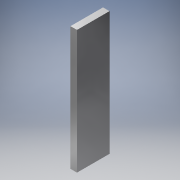
# Autodesk Inventor part: frame_front
Saved by Autodesk Inventor 2018 (Build 220112000, 112)
## iProperties
Created: 2018-05-23
Part Number: frame_front
Material: アルミニウム 6061
Document SubType Name: Sheet Metal
Designer: NaMACHAN
Density: 2.7 g/cm^3
Sheet Metal Rule: 2mmAl
Appearance: アルミニウム - フラット
Author: NaMACHAN
Autodesk Inventor part; units mm, degrees
ref_plane "YZ Plane" through (0, 0, 0) normal (1, 0, 0) x (0, 1, 0)
ref_plane "XZ Plane" through (0, 0, 0) normal (0, 1, 0) x (-1, 0, 0)
ref_plane "XY Plane" through (0, 0, 0) normal (0, 0, 1) x (1, 0, 0)
sketch "スケッチ1" plane through (0, 0, 0) normal (1, 0, 0) x (0, 1, 0)
  line L0 (0, 0) -> (0, -38)
  line L1 (0, -38) -> (-10, -38)
  line L2 (-10, -38) -> (-10, 0)
  line L3 (-10, 0) -> (0, 0)
  dimension "d0" = 38
  dimension "d2" = 10
  measures "d0" distance of L0.start L0.end
  measures "d2" distance of L0.end L1.end
extrude "プレート1" add sketch "スケッチ1" along normal blind 2
sketch "スケッチ14" plane through (-2, 2, -38) normal (0, 1, 0) x (-1, 0, 0)
  line L0 (0, 38) -> (0, 0)
  line L1 (0, 0) -> (8, 0)
  line L2 (8, 0) -> (8, 38)
  line L3 (8, 38) -> (0, 38)
  constraints: 6 end point, 1 horizontal, 1 perpendicular, 1 vertical
edge flange "フランジ1" height 12 angle 90 thickness 2 bend radius 2 thickness toward (0, 1, 0) relief tear relief width 2 relief depth 1 edges at (0, 0, -19) wall of the first edge with corners at (-2, 2, 0) (-2, 2, -38) (-10, 2, -38) (-10, 2, 0)
bend "曲げ26"
corner "コーナー1"
sketch "スケッチ15" plane through (-2, -12, 0) normal (0, -1, 0) x (1, 0, 0)
  line L0 (0, -38) -> (0, 0)
  line L1 (0, 0) -> (-8, 0)
  line L2 (-8, 0) -> (-8, -38)
  line L3 (-8, -38) -> (0, -38)
  constraints: 6 end point, 1 horizontal, 1 perpendicular, 1 vertical
edge flange "フランジ2" height 12 angle 90 thickness 2 bend radius 2 thickness toward (0, -1, 0) relief tear relief width 2 relief depth 1 edges at (0, -10, -19) wall of the first edge with corners at (-2, -12, -38) (-2, -12, 0) (-10, -12, 0) (-10, -12, -38)
bend "曲げ27"
corner "コーナー2"
sketch "スケッチ16" plane through (-10, 4, 0) normal (0, 1, 0) x (1, 0, 0)
  line L0 (5.5, 4) -> (5.5, 34)
  arc A0 (5.5, 34) -> (2.5, 34) centre (4, 34) ccw
  line L1 (2.5, 34) -> (2.5, 4)
  arc A1 (2.5, 4) -> (5.5, 4) centre (4, 4) ccw
  line L2 (0, 38) -> (8, 38) projected
  line L3 (8, 0) -> (0, 0) projected
  point P0 (10, 0)
  point P1 (4, 38)
  dimension "d192" = 1.5
  dimension "d193" = 4
  dimension "d194" = 4
  constraints: 4 end point, 4 point on circle, 4 tangent, 2 centre point, 1 midpoint, 1 parallel, 1 vertical, 1 vertical alignment
  measures "d192" radius of A0
  measures "d193" distance from line of L2 A0.centre
  measures "d194" distance from line of L3 A1.centre
extrude "押し出し1" cut sketch "スケッチ16" against normal blind 10
sketch "スケッチ17" plane through (-10, -12, 0) normal (0, 1, 0) x (1, 0, 0)
  line L0 (0, 0) -> (8, 0) projected
  line L1 (0, 38) -> (8, 38) projected
  point P0 (10, 0)
  point P1 (4, 5)
  point P2 (4, 33)
  point P3 (4, 0)
  point P4 (4, 38)
  dimension "d197" = 5
  dimension "d198" = 5
  constraints: 2 midpoint, 2 vertical alignment
  measures "d197" distance from line of L0 point (4, 5)
  measures "d198" distance from line of L1 point (4, 33)
hole "穴1" at (-6, -12, -5) at (-6, -12, -33) direction (0, -1, 0) diameter 3 end through all
equation "\"d204\" = Thickness"
equation "\"d3\" = Thickness"
equation "\"d172\" = BendReliefWidth"
equation "\"d173\" = BendReliefDepth"
equation "\"d174\" = MinimumRemnant"
equation "\"d175\" = TransitionRadius"
equation "\"d178\" = BendRadius"
equation "\"d179\" = CornerReliefSize"
equation "\"d180\" = GapSize"
equation "\"d181\" = JacobiRadiusSize"
equation "\"d182\" = BendReliefWidth"
equation "\"d183\" = BendReliefDepth"
equation "\"d184\" = MinimumRemnant"
equation "\"d185\" = TransitionRadius"
equation "\"d188\" = BendRadius"
equation "\"d189\" = CornerReliefSize"
equation "\"d190\" = GapSize"
equation "\"d191\" = JacobiRadiusSize"
equation "\"BendRadius\" = Thickness"
equation "\"BendReliefWidth\" = Thickness"
equation "\"BendReliefDepth\" = 0.5 * Thickness"
equation "\"CornerReliefSize\" = 4 * Thickness"
equation "\"MinimumRemnant\" = 2 * Thickness"
equation "\"TransitionRadius\" = BendRadius"
equation "\"JacobiRadiusSize\" = BendRadius"
equation "\"GapSize\" = Thickness"
equation "\"Thickness\" = 2"
